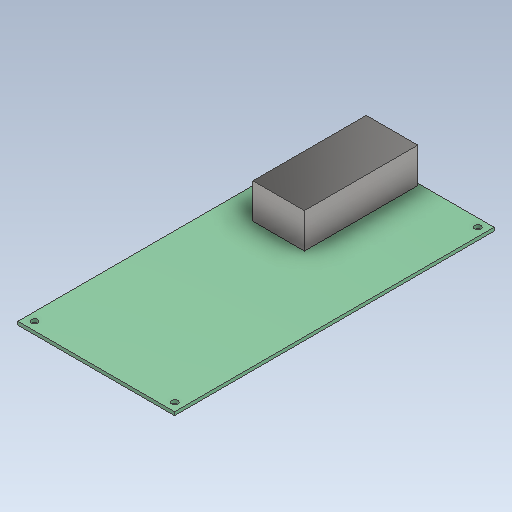
# Autodesk Inventor part: Coms Board V1
Saved by Autodesk Inventor 2021 (Build 250183000, 183)
## iProperties
Created: 2020-07-06
Part Number: Coms Board V1
Material: Generic
Document SubType Name: Modeling
Designer: jgray
Density: 1 g/cm^3
Appearance: Default
Author: jgray
Autodesk Inventor part; units mm, degrees
ref_plane "YZ Plane" through (0, 0, 0) normal (1, 0, 0) x (0, 1, 0)
ref_plane "XZ Plane" through (0, 0, 0) normal (0, 1, 0) x (-1, 0, 0)
ref_plane "XY Plane" through (0, 0, 0) normal (0, 0, 1) x (1, 0, 0)
sketch "Sketch1" plane through (0, 0, 0) normal (0, 1, 0) x (-1, 0, 0)
  line L0 (0, 0) -> (76, 0)
  line L1 (76, 0) -> (76, -155)
  line L2 (76, -155) -> (0, -155)
  line L3 (0, -155) -> (0, 0)
  line L4 (81.1574, -77.5) -> (-13.3813, -77.5) construction
  line L5 (38, 8.4809) -> (38, -161.1275) construction
  line L6 (4, -151) -> (72, -151) construction
  line L7 (72, -151) -> (72, -4) construction
  line L8 (72, -4) -> (4, -4) construction
  line L9 (4, -4) -> (4, -151) construction
  line L10 (4, -151) -> (72, -4) construction
  line L11 (72, -151) -> (4, -4) construction
  circle A0 centre (72, -4) radius 1.55
  circle A1 centre (72, -151) radius 1.55
  circle A2 centre (4, -151) radius 1.55
  circle A3 centre (4, -4) radius 1.55
  point P0 (76, -77.5)
  point P1 (38, -155)
  point P2 (38, -77.5)
  dimension "d0" = 76
  dimension "d1" = 155
  dimension "d2" = 68
  dimension "d3" = 147
  dimension "d4" = 3.1
  dimension "d5" = 3.1
  dimension "d6" = 3.1
  dimension "d7" = 3.1
  constraints: 24 end point, 4 centre point, 4 coincident, 4 midpoint, 4 parallel, 4 point on line, 3 horizontal, 2 perpendicular, 1 vertical
  measures "d0" distance of L1.end L2.end
  measures "d1" distance of L0.end L1.end
  measures "d2" distance of L8.end L7.end
  measures "d3" distance of L7.end L6.end
  measures "d4" diameter of A0
  measures "d5" diameter of A1
  measures "d6" diameter of A2
  measures "d7" diameter of A3
extrude "Extrusion1" add sketch "Sketch1" against normal blind 1.65
sketch "Sketch2" plane through (0, 0, 0) normal (0, 1, 0) x (1, 0, 0)
  line L0 (-61, 99) -> (-36, 99)
  line L1 (-36, 99) -> (-36, 154)
  line L2 (-36, 154) -> (-61, 154)
  line L3 (-61, 154) -> (-61, 99)
  line L4 (0, 155) -> (-76, 155) projected
  line L5 (-76, 155) -> (-76, 0) projected
  point P0 (0, 0)
  dimension "d10" = 25
  dimension "d11" = 55
  dimension "d12" = 56
  dimension "d13" = 40
  constraints: 8 end point, 2 parallel, 1 horizontal, 1 perpendicular
  measures "d10" distance of L2.end L1.end
  measures "d11" distance of L1.end L0.end
  measures "d12" distance from line of L4 L0.start
  measures "d13" distance between parallel lines of L5 L1
extrude "Extrusion2" add sketch "Sketch2" along normal blind 17
body "Solid1"
